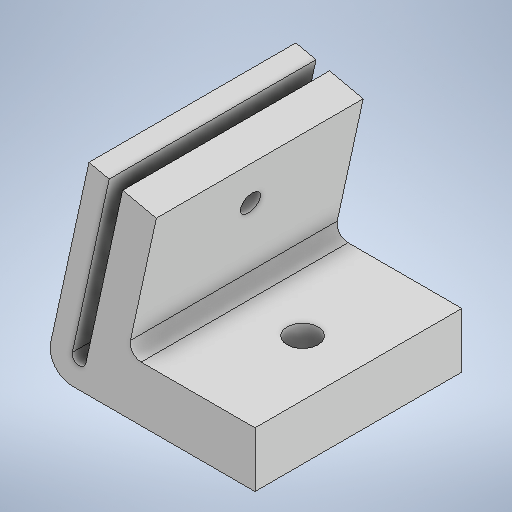
# Autodesk Inventor part: lustereczko
Saved by Autodesk Inventor 2025.1 (Build 291241000, 241)
## iProperties
Created: 2024-10-30
Part Number: lustereczko
Material: Ogólny
Document SubType Name: Modeling
Designer: PC
Density: 1 g/cm^3
Appearance: Domyślna
Author: PC
Autodesk Inventor part; units mm, degrees
ref_plane "YZ Plane" through (0, 0, 0) normal (1, 0, 0) x (0, 1, 0)
ref_plane "XZ Plane" through (0, 0, 0) normal (0, 1, 0) x (-1, 0, 0)
ref_plane "XY Plane" through (0, 0, 0) normal (0, 0, 1) x (1, 0, 0)
sketch "Szkic1" plane through (0, 0, 0) normal (0, 0, 1) x (1, 0, 0)
  line L0 (0, -6.7527) -> (0, 35.3194) projected
  line L1 (0.8414, 3.8525) -> (6.4011, 29.3091)
  line L2 (6.4011, 29.3091) -> (9.3321, 28.669)
  line L3 (9.3321, 28.669) -> (3.9978, 4.2447)
  line L4 (5.9517, 3.818) -> (11.286, 28.2423)
  line L5 (11.286, 28.2423) -> (16.1709, 27.1754)
  arc A0 (3.9978, 4.2447) -> (5.9517, 3.818) centre (4.9747, 4.0314) ccw
  line L6 (16.1709, 27.1754) -> (12.4071, 9.942)
  line L7 (13.9707, 8) -> (30.48, 8)
  arc A1 (12.4071, 9.942) -> (13.9707, 8) centre (13.9707, 9.6005) ccw
  line L8 (3.9433, 0) -> (30.48, 0)
  line L9 (30.48, 0) -> (30.48, 8)
  arc A2 (0.8414, 3.8525) -> (3.9433, 0) centre (3.9433, 3.175) ccw
  point P0 (0, 0)
  dimension "d0" = 12.32
  dimension "d1" = 3
  dimension "d2" = 30
  dimension "d3" = 5
  dimension "d4" = 8
  dimension "d5" = 25
  dimension "d6" = 2
  dimension "d7" = 30.48
  dimension "d8" = 1.6005
  dimension "d9" = 3.175
  constraints: 18 end point, 6 point on circle, 6 tangent, 3 centre point, 3 perpendicular, 2 horizontal, 2 parallel, 2 point on line, 1 collinear
  measures "d0" angle of L0 L1
  measures "d1" distance of L1.end L2.end
  measures "d2" distance of point (0, 0) L1.end
  measures "d3" distance of L4.end L5.end
  measures "d4" distance from line of point (0, 0) L7
  measures "d5" distance of L4.start L4.end
  measures "d6" distance between parallel lines of L4 L3
  measures "d7" distance from line of point (0, 0) L9
  measures "d8" radius of A1
  measures "d9" radius of A2
extrude "Wyciągnięcie proste1" add sketch "Szkic1" along normal blind 30
sketch "Szkic2" plane through (13.9707, 8, 0) normal (0, 1, 0) x (1, 0, 0)
  circle A0 centre (8.4108, -15) radius 2.25
  point P0 (-13.9707, 0)
  dimension "d12" = 4.5
  constraints: 1 centre point
  measures "d12" diameter of A0
extrude "Wyciągnięcie proste2" cut sketch "Szkic2" against normal blind 30
sketch "Szkic3" plane through (16.1709, 27.1754, 30) normal (0.9769712, -0.2133714, 0) x (0, 0, -1)
  circle A0 centre (15, -6.4184) radius 1.45
  point P0 (30, -30)
  dimension "d15" = 2.9
  constraints: 1 centre point
  measures "d15" diameter of A0
extrude "Wyciągnięcie proste3" cut sketch "Szkic3" against normal up to next
